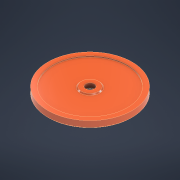
# Autodesk Inventor part: 009
Saved by Autodesk Inventor 2022 (Build 260153000, 153)
## iProperties
Created: 2021-10-31
Part Number: 009
Material: Stainless Steel, 440C
Document SubType Name: Modeling
Designer: vinicius.miguel
Density: 7.75 g/cm^3
Appearance: Smooth - Light Orange
Author: vinicius.miguel
Autodesk Inventor part; units mm, degrees
ref_plane "YZ Plane" through (0, 0, 0) normal (1, 0, 0) x (0, 1, 0)
ref_plane "XZ Plane" through (0, 0, 0) normal (0, 1, 0) x (-1, 0, 0)
ref_plane "XY Plane" through (0, 0, 0) normal (0, 0, 1) x (1, 0, 0)
sketch "Sketch1" plane through (0, 0, 0) normal (0, 0, 1) x (1, 0, 0)
  line L0 (-39, 0) -> (-34.5, 0)
  line L1 (-34.5, 0) -> (-34.5, 1)
  line L2 (-34.5, 1) -> (-4, 1)
  line L3 (-4, 1) -> (-4, 6)
  line L4 (-4, 6) -> (-8, 6)
  line L5 (-8, 6) -> (-8, 5)
  line L6 (-8, 5) -> (-34.5, 5)
  line L7 (-34.5, 5) -> (-34.5, 6)
  line L8 (-34.5, 6) -> (-39, 6)
  line L9 (-39, 6) -> (-39, 0)
  line L10 (0, 0) -> (0, 3.3453)
  line L11 (-34.5, 1) -> (-34.5, 1.25)
  line L12 (-34.5, 1.25) -> (-32.5, 1)
  dimension "d0" = 8
  dimension "d3" = 16
  dimension "d8" = 1
  dimension "d9" = 1
  dimension "d10" = 4
  dimension "d11" = 78
  dimension "d18" = 69
  dimension "d23" = 0.25
  dimension "d24" = 2
  constraints: 26 end point, 8 perpendicular, 3 point on line, 2 vertical, 1 horizontal, 1 horizontal alignment, 1 vertical alignment
  measures "d0" diameter of L3 L10
  measures "d3" diameter of L4.end L10
  measures "d8" distance of L6.end L7.end
  measures "d9" distance of L0.end L1.end
  measures "d10" distance between parallel lines of L2 L6
  measures "d11" diameter of L9 L10
  measures "d18" diameter of L1 L10
  measures "d23" distance of L1.end L11.end
  measures "d24" distance from line of L12.end L11
revolve "Revolution1" add sketch "Sketch1" angle 360 about axis through (0, 0, 0) along (0, 1, 0)
chamfer "Chamfer1" distance 1 angle 45 2 edges at (4, 1, 0) (8, 5, 0)
chamfer "Chamfer2" distance 0.5 angle 45 1 edges at (39, 0, 0)
body "Solid1"
